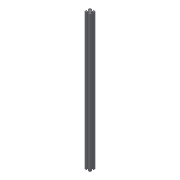
# Autodesk Inventor part: Propile_202050
Saved by Autodesk Inventor 2019 (Build 230136000, 136)
## iProperties
Created: 2019-05-03
Part Number: Propile_202050
Material: 일반
Document SubType Name: Modeling
Designer: hinmo
Density: 1 g/cm^3
Appearance: 기본값
Author: hinmo
Autodesk Inventor part; units mm, degrees
ref_plane "YZ Plane" through (0, 0, 0) normal (1, 0, 0) x (0, 1, 0)
ref_plane "XZ Plane" through (0, 0, 0) normal (0, 1, 0) x (-1, 0, 0)
ref_plane "XY Plane" through (0, 0, 0) normal (0, 0, 1) x (1, 0, 0)
sketch "스케치1" plane through (0, 0, 0) normal (0, 1, 0) x (-1, 0, 0)
  circle A0 centre (-26.5671, -74.7948) radius 2.15 projected
  circle A1 centre (-19.5671, -81.7948) radius 2 projected
  circle A2 centre (-19.5671, -67.7948) radius 2 projected
  circle A3 centre (-33.5671, -67.7948) radius 2 projected
  circle A4 centre (-33.5671, -81.7948) radius 2 projected
  arc A5 (-29.2171, -65.0948) -> (-29.5171, -64.7948) centre (-29.5171, -65.0948) ccw projected
  line L0 (-29.5171, -64.7948) -> (-36.2671, -64.7948) projected
  arc A6 (-36.2671, -64.7948) -> (-36.5671, -65.0948) centre (-36.2671, -65.0948) ccw projected
  line L1 (-36.5671, -65.0948) -> (-36.5671, -71.8448) projected
  arc A7 (-36.5671, -71.8448) -> (-36.2671, -72.1448) centre (-36.2671, -71.8448) ccw projected
  line L2 (-36.2671, -72.1448) -> (-35.0671, -72.1448) projected
  line L3 (-35.0671, -72.1448) -> (-35.0671, -70.6448) projected
  line L4 (-35.0671, -70.6448) -> (-31.5671, -70.6448) projected
  arc A8 (-31.5671, -78.9448) -> (-31.5671, -70.6448) centre (-36.8271, -74.7948) ccw projected
  line L5 (-31.5671, -78.9448) -> (-35.0671, -78.9448) projected
  line L6 (-35.0671, -78.9448) -> (-35.0671, -77.4448) projected
  line L7 (-35.0671, -77.4448) -> (-36.2671, -77.4448) projected
  arc A9 (-36.2671, -77.4448) -> (-36.5671, -77.7448) centre (-36.2671, -77.7448) ccw projected
  line L8 (-36.5671, -77.7448) -> (-36.5671, -84.4948) projected
  arc A10 (-36.5671, -84.4948) -> (-36.2671, -84.7948) centre (-36.2671, -84.4948) ccw projected
  line L9 (-36.2671, -84.7948) -> (-29.5171, -84.7948) projected
  arc A11 (-29.5171, -84.7948) -> (-29.2171, -84.4948) centre (-29.5171, -84.4948) ccw projected
  line L10 (-29.2171, -84.4948) -> (-29.2171, -83.2948) projected
  line L11 (-29.2171, -83.2948) -> (-30.7171, -83.2948) projected
  line L12 (-30.7171, -83.2948) -> (-30.7171, -79.7948) projected
  arc A12 (-22.4171, -79.7948) -> (-30.7171, -79.7948) centre (-26.5671, -85.0548) ccw projected
  line L13 (-22.4171, -79.7948) -> (-22.4171, -83.2948) projected
  line L14 (-22.4171, -83.2948) -> (-23.9171, -83.2948) projected
  line L15 (-23.9171, -83.2948) -> (-23.9171, -84.4948) projected
  arc A13 (-23.9171, -84.4948) -> (-23.6171, -84.7948) centre (-23.6171, -84.4948) ccw projected
  line L16 (-23.6171, -84.7948) -> (-16.8671, -84.7948) projected
  arc A14 (-16.8671, -84.7948) -> (-16.5671, -84.4948) centre (-16.8671, -84.4948) ccw projected
  line L17 (-16.5671, -84.4948) -> (-16.5671, -77.7448) projected
  arc A15 (-16.5671, -77.7448) -> (-16.8671, -77.4448) centre (-16.8671, -77.7448) ccw projected
  line L18 (-16.8671, -77.4448) -> (-18.0671, -77.4448) projected
  line L19 (-18.0671, -77.4448) -> (-18.0671, -78.9448) projected
  line L20 (-18.0671, -78.9448) -> (-21.5671, -78.9448) projected
  arc A16 (-21.5671, -70.6448) -> (-21.5671, -78.9448) centre (-16.3071, -74.7948) ccw projected
  line L21 (-21.5671, -70.6448) -> (-18.0671, -70.6448) projected
  line L22 (-18.0671, -70.6448) -> (-18.0671, -72.1448) projected
  line L23 (-18.0671, -72.1448) -> (-16.8671, -72.1448) projected
  arc A17 (-16.8671, -72.1448) -> (-16.5671, -71.8448) centre (-16.8671, -71.8448) ccw projected
  line L24 (-16.5671, -71.8448) -> (-16.5671, -65.0948) projected
  arc A18 (-16.5671, -65.0948) -> (-16.8671, -64.7948) centre (-16.8671, -65.0948) ccw projected
  line L25 (-16.8671, -64.7948) -> (-23.6171, -64.7948) projected
  arc A19 (-23.6171, -64.7948) -> (-23.9171, -65.0948) centre (-23.6171, -65.0948) ccw projected
  line L26 (-23.9171, -65.0948) -> (-23.9171, -66.2948) projected
  line L27 (-23.9171, -66.2948) -> (-22.4171, -66.2948) projected
  line L28 (-22.4171, -66.2948) -> (-22.4171, -69.7948) projected
  arc A20 (-30.7171, -69.7948) -> (-22.4171, -69.7948) centre (-26.5671, -64.5348) ccw projected
  line L29 (-30.7171, -69.7948) -> (-30.7171, -66.2948) projected
  line L30 (-30.7171, -66.2948) -> (-29.2171, -66.2948) projected
  line L31 (-29.2171, -66.2948) -> (-29.2171, -65.0948) projected
  circle A21 centre (0, 0) radius 2.15
  circle A22 centre (7, -7) radius 2
  circle A23 centre (7, 7) radius 2
  circle A24 centre (-7, 7) radius 2
  circle A25 centre (-7, -7) radius 2
  arc A26 (-2.65, 9.7) -> (-2.95, 10) centre (-2.95, 9.7) ccw
  line L32 (-2.95, 10) -> (-9.7, 10)
  arc A27 (-9.7, 10) -> (-10, 9.7) centre (-9.7, 9.7) ccw
  line L33 (-10, 9.7) -> (-10, 2.95)
  arc A28 (-10, 2.95) -> (-9.7, 2.65) centre (-9.7, 2.95) ccw
  line L34 (-9.7, 2.65) -> (-8.5, 2.65)
  line L35 (-8.5, 2.65) -> (-8.5, 4.15)
  line L36 (-8.5, 4.15) -> (-5, 4.15)
  arc A29 (-5, -4.15) -> (-5, 4.15) centre (-10.26, 0) ccw
  line L37 (-5, -4.15) -> (-8.5, -4.15)
  line L38 (-8.5, -4.15) -> (-8.5, -2.65)
  line L39 (-8.5, -2.65) -> (-9.7, -2.65)
  arc A30 (-9.7, -2.65) -> (-10, -2.95) centre (-9.7, -2.95) ccw
  line L40 (-10, -2.95) -> (-10, -9.7)
  arc A31 (-10, -9.7) -> (-9.7, -10) centre (-9.7, -9.7) ccw
  line L41 (-9.7, -10) -> (-2.95, -10)
  arc A32 (-2.95, -10) -> (-2.65, -9.7) centre (-2.95, -9.7) ccw
  line L42 (-2.65, -9.7) -> (-2.65, -8.5)
  line L43 (-2.65, -8.5) -> (-4.15, -8.5)
  line L44 (-4.15, -8.5) -> (-4.15, -5)
  arc A33 (4.15, -5) -> (-4.15, -5) centre (0, -10.26) ccw
  line L45 (4.15, -5) -> (4.15, -8.5)
  line L46 (4.15, -8.5) -> (2.65, -8.5)
  line L47 (2.65, -8.5) -> (2.65, -9.7)
  arc A34 (2.65, -9.7) -> (2.95, -10) centre (2.95, -9.7) ccw
  line L48 (2.95, -10) -> (9.7, -10)
  arc A35 (9.7, -10) -> (10, -9.7) centre (9.7, -9.7) ccw
  line L49 (10, -9.7) -> (10, -2.95)
  arc A36 (10, -2.95) -> (9.7, -2.65) centre (9.7, -2.95) ccw
  line L50 (9.7, -2.65) -> (8.5, -2.65)
  line L51 (8.5, -2.65) -> (8.5, -4.15)
  line L52 (8.5, -4.15) -> (5, -4.15)
  arc A37 (5, 4.15) -> (5, -4.15) centre (10.26, 0) ccw
  line L53 (5, 4.15) -> (8.5, 4.15)
  line L54 (8.5, 4.15) -> (8.5, 2.65)
  line L55 (8.5, 2.65) -> (9.7, 2.65)
  arc A38 (9.7, 2.65) -> (10, 2.95) centre (9.7, 2.95) ccw
  line L56 (10, 2.95) -> (10, 9.7)
  arc A39 (10, 9.7) -> (9.7, 10) centre (9.7, 9.7) ccw
  line L57 (9.7, 10) -> (2.95, 10)
  arc A40 (2.95, 10) -> (2.65, 9.7) centre (2.95, 9.7) ccw
  line L58 (2.65, 9.7) -> (2.65, 8.5)
  line L59 (2.65, 8.5) -> (4.15, 8.5)
  line L60 (4.15, 8.5) -> (4.15, 5)
  arc A41 (-4.15, 5) -> (4.15, 5) centre (0, 10.26) ccw
  line L61 (-4.15, 5) -> (-4.15, 8.5)
  line L62 (-4.15, 8.5) -> (-2.65, 8.5)
  line L63 (-2.65, 8.5) -> (-2.65, 9.7)
  constraints: 64 end point, 32 point on circle, 21 centre point
extrude "돌출1" add sketch "스케치1" along normal blind 500 contours L63 L62 L61 A41 L60 L59 L58 A40 L57 A39 L56 A38 L55 L54 L53 A37 L52 L51 L50 A36 L49 A35 L48 A34 L47 L46 L45 A33 L44 L43 L42 A32 L41 A31 L40 A30 L39 L38 L37 A29 L36 L35 L34 A28 L33 A27 L32 A26
